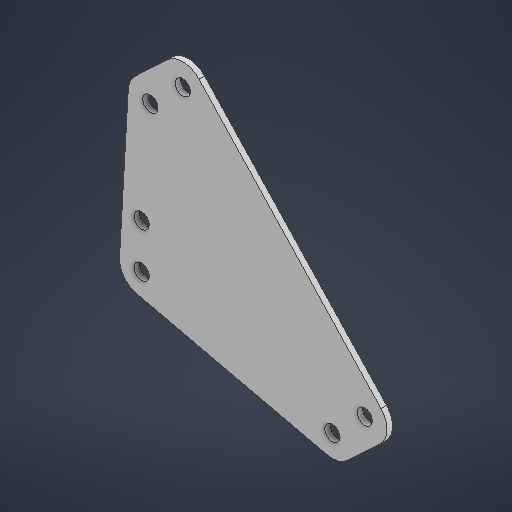
# Autodesk Inventor part: 2-Gearbox
Saved by Autodesk Inventor 2026.1 (Build 301233000, 233)
## iProperties
Created: 2025-08-06
Part Number: 2-Gearbox
Material: Generic
Document SubType Name: Modeling
Designer: roejo
Density: 1 g/cm^3
Appearance: Default
Author: roejo
Autodesk Inventor part; units mm, degrees
ref_plane "YZ Plane" through (0, 0, 0) normal (1, 0, 0) x (0, 1, 0)
ref_plane "XZ Plane" through (0, 0, 0) normal (0, 1, 0) x (-1, 0, 0)
ref_plane "XY Plane" through (0, 0, 0) normal (0, 0, 1) x (1, 0, 0)
sketch "Sketch1" plane through (0, 0, 0) normal (0, 0, 1) x (1, 0, 0)
  circle A0 centre (58.7079, -22.221) radius 2.1844
  circle A1 centre (67.9751, -13.5372) radius 2.1844
  circle A2 centre (4.1043, 3.1638) radius 2.1844
  circle A3 centre (4.1043, -9.5362) radius 2.1844
  circle A4 centre (15.8718, 42.0658) radius 2.1844
  circle A5 centre (6.6046, 33.3819) radius 2.1844
  circle A6 centre (6.6046, 33.3819) radius 6.35
  circle A7 centre (15.8718, 42.0658) radius 6.35
  circle A8 centre (4.1043, -9.5362) radius 6.35
  circle A9 centre (58.7079, -22.221) radius 6.35
  circle A10 centre (67.9751, -13.5372) radius 6.35
  line L0 (20.5054, 46.4077) -> (72.6087, -9.1952)
  line L1 (72.317, -18.1707) -> (63.0499, -26.8546)
  line L2 (2.6674, -15.7215) -> (57.2711, -28.4063)
  line L3 (0.2654, 33.7512) -> (-2.235, -9.1669)
  line L4 (2.2627, 38.0155) -> (11.5299, 46.6994)
  dimension "d8" = 12.7
  dimension "d9" = 12.7
  dimension "d10" = 12.7
  dimension "d11" = 12.7
  dimension "d12" = 12.7
  constraints: 11 centre point, 10 end point, 10 point on circle, 8 tangent, 5 coincident, 1 parallel, 1 perpendicular, 5 other
  measures "d8" diameter of A6
  measures "d9" diameter of A7
  measures "d10" diameter of A8
  measures "d11" diameter of A9
  measures "d12" diameter of A10
extrude "Extrusion1" add sketch "Sketch1" along normal blind 1.5875
body "Solid1"
